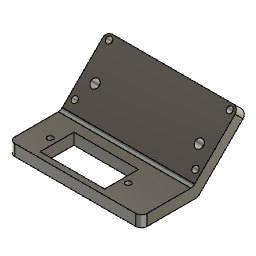
SOAR_Sensor_Holder-v2 (Autodesk Fusion 360 design; units mm, degrees)
Autodesk Fusion 360 part; units mm, degrees
sketch "Sketch1" plane through (0, 0, 0) normal (0, 0, 1) x (1, 0, 0)
  line L0 (0, 0) -> (47, 0)
  line L1 (47, 0) -> (47, 20)
  line L2 (47, 20) -> (0, 20)
  line L3 (0, 20) -> (0, 0)
  line L4 (0, 20) -> (47, 20)
  line L5 (47, 20) -> (47, 16)
  line L6 (47, 16) -> (0, 16)
  line L7 (0, 16) -> (0, 20)
  line L8 (4.25, 14) -> (36.75, 14)
  line L9 (36.75, 14) -> (36.75, 2)
  line L10 (36.75, 2) -> (4.25, 2)
  line L11 (4.25, 2) -> (4.25, 14)
  line L12 (4.25, 2) -> (9.05, 2)
  line L13 (9.05, 2) -> (9.05, 14)
  line L14 (9.05, 14) -> (4.25, 14)
  line L15 (4.25, 14) -> (4.25, 2)
  line L16 (36.75, 2) -> (31.95, 2)
  line L17 (31.95, 2) -> (31.95, 14)
  line L18 (31.95, 14) -> (36.75, 14)
  line L19 (36.75, 14) -> (36.75, 2)
  circle A0 centre (6.65, 8) radius 1
  circle A1 centre (34.35, 8) radius 1
  dimension "d1" = 47
  dimension "d2" = 20
  dimension "d5" = 4
  dimension "d20" = 32.5
  dimension "d21" = 12
  dimension "d22" = 4.8
  dimension "d23" = 4.8
  dimension "d24" = 2
  dimension "d25" = 2
  constraint horizontal L0
  constraint vertical L1
  constraint horizontal L2
  constraint vertical L3
  constraint coincident L0.start L3.end
  constraint horizontal L4
  constraint vertical L5
  constraint horizontal L6
  constraint vertical L7
  constraint horizontal L8
  constraint vertical L9
  constraint horizontal L10
  constraint vertical L11
  constraint horizontal L12
  constraint vertical L13
  constraint horizontal L14
  constraint vertical L15
  constraint coincident L8 L13.end
  constraint horizontal L16
  constraint vertical L17
  constraint horizontal L18
  constraint vertical L19
  measures "d1" distance of L0.start L0.end
  measures "d2" distance of L0.start L2.end
  measures "d5" distance of L2.end L6.end
  measures "d20" distance of L8.start L8.end
  measures "d21" distance of L8.start L10.end
  measures "d22" distance of L10.end L12.end
  measures "d23" distance of L9.end L16.end
  measures "d24" diameter of A0
  measures "d25" diameter of A1
extrude "Extrude1" add sketch "Sketch1" along normal blind 4 contours L0 L1 L3 L6 | L8 L10 L11 L12 L13 L14 L15 | L8 L9 L10 L16 L17 L18 L19 makes body 1
extrude "Extrude6" add sketch "Sketch1" along normal blind 4 contours L1 L2 L3 L4 L5 L6 L7 bodies 1
extrude "Extrude2" add sketch "Sketch1" along normal blind 24.7 separate body contours L1 L2 L3 L4 L5 L6 L7 makes body 2
sketch "Sketch2" plane through (0, 16, 0) normal (0, -1, 0) x (1, 0, 0)
  circle A0 centre (2.09, 23) radius 0.8
  line L0 (46.21, 24.3) -> (46.21, 3.96)
  circle A1 centre (2.09, 5.76) radius 1.2
  circle A2 centre (44.91, 23) radius 0.8
  circle A3 centre (44.91, 23) radius 1.2
  line L1 (46.21, 3.96) -> (0.79, 3.96)
  circle A4 centre (2.09, 23) radius 1.2
  circle A5 centre (44.91, 5.76) radius 1.2
  line L2 (0.79, 24.3) -> (46.21, 24.3)
  circle A6 centre (2.09, 5.76) radius 0.8
  line L3 (0.79, 3.96) -> (0.79, 24.3)
  circle A7 centre (44.91, 5.76) radius 0.8
hole "Hole1" at (2.09, 16, 23) direction (0, 1, 0) diameter 2.1 depth 4 tip angle 180 bodies 1 2
hole "Hole2" at (44.91, 16, 23) direction (0, 1, 0) diameter 2.1 depth 4 tip angle 180 bodies 2 1
hole "Hole3" at (44.91, 16, 5.76) direction (0, 1, 0) diameter 2.1 depth 4 tip angle 180 bodies 1 2
hole "Hole4" at (2.09, 16, 5.76) direction (0, 1, 0) diameter 2.1 depth 4 tip angle 180 bodies 2 1
sketch "Sketch3" plane through (0, 16, 0) normal (0, -1, 0) x (1, 0, 0)
  line L0 (47, 0) -> (47, 24.7)
  line L1 (47, 24.7) -> (0, 24.7)
  line L2 (0, 24.7) -> (0, 0)
  line L3 (38.25, 18.548) -> (27.5, 18.548)
  line L4 (8.75, 5.548) -> (38.25, 5.548)
  circle A0 centre (5, 11.8211) radius 1.6
  line L5 (8.75, 7.848) -> (8.75, 5.548)
  line L6 (5, 8.0711) -> (6.15, 8.0711)
  line L7 (8.75, 16.248) -> (8.75, 7.848)
  line L8 (38.25, 8.0711) -> (40.85, 8.0711)
  line L9 (19.5, 18.548) -> (8.75, 18.548)
  line L10 (40.85, 15.5711) -> (38.25, 15.5711)
  line L11 (42, 8.0711) -> (40.85, 8.0711)
  line L12 (38.25, 16.248) -> (38.25, 18.548)
  circle A1 centre (42, 11.8211) radius 1.6
  line L13 (8.75, 8.0711) -> (6.15, 8.0711)
  line L14 (27.5, 18.548) -> (19.5, 18.548)
  line L15 (8.75, 18.548) -> (8.75, 16.248)
  line L16 (38.25, 7.848) -> (38.25, 16.248)
  line L17 (40.85, 15.5711) -> (42, 15.5711)
  line L18 (6.15, 15.5711) -> (5, 15.5711)
  line L19 (6.15, 15.5711) -> (8.75, 15.5711)
  line L20 (38.25, 5.548) -> (38.25, 7.848)
  arc A2 (5, 15.5711) -> (5, 8.0711) centre (5, 11.8211) ccw
  arc A3 (42, 8.0711) -> (42, 15.5711) centre (42, 11.8211) ccw
  circle A4 centre (2.09, 5.76) radius 1.05
  circle A5 centre (44.91, 5.76) radius 1.05
  circle A6 centre (2.09, 23) radius 1.05
  circle A7 centre (44.91, 23) radius 1.05
  line L21 (0, 0) -> (47, 0)
hole "Hole5" at (42, 16, 11.8211) direction (0, 1, 0) diameter 3 depth 4 tip angle 180 bodies 2 1
hole "Hole6" at (5, 16, 11.8211) direction (0, 1, 0) diameter 3 depth 4 tip angle 180 bodies 1 2
move_body "Move1" bodies 2 to x (1, 0, 0) y (0, 0.707107, -0.707107) z (0, 0.707107, 0.707107) at (0, 5.8579, 14.1421)
combine "Combine1" operation add target body 1 tool bodies 2
fillet "Fillet2" radius 2 6 edges at (23.5, 20, 0) (23.5, 18.3431, 4) (47, 36.0513, 18.8798) (0, 36.0513, 18.8798) (0, 0, 2) (47, 0, 2) on bodies 1
